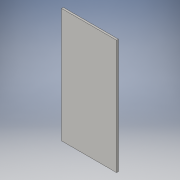
# Autodesk Inventor part: RaspberryBox_Backplate
Saved by Autodesk Inventor 2016 (Build 200138000, 138)
## iProperties
Created: 2016-12-27
Part Number: RaspberryBox_Backplate
Material: Generisch
Document SubType Name: Modeling
Designer: Moritz
Density: 1 g/cm^3
Appearance: Vorgabe
Author: Moritz
Autodesk Inventor part; units mm, degrees
ref_plane "YZ Plane" through (0, 0, 0) normal (1, 0, 0) x (0, 1, 0)
ref_plane "XZ Plane" through (0, 0, 0) normal (0, 1, 0) x (-1, 0, 0)
ref_plane "XY Plane" through (0, 0, 0) normal (0, 0, 1) x (1, 0, 0)
sketch "Skizze1" plane through (0, 0, 0) normal (0, 1, 0) x (-1, 0, 0)
  line L0 (-44, 91.5) -> (44, 91.5)
  line L1 (44, 91.5) -> (44, -91.5)
  line L2 (44, -91.5) -> (-44, -91.5)
  line L3 (-44, -91.5) -> (-44, 91.5)
  line L4 (-44, 91.5) -> (44, -91.5) construction
  line L5 (44, 91.5) -> (-44, -91.5) construction
  point P0 (0, 0)
  dimension "d0" = 88
  dimension "d1" = 183
  constraints: 12 end point, 2 midpoint, 2 parallel, 1 horizontal, 1 perpendicular
  measures "d0" distance of L1.end L2.end
  measures "d1" distance of L0.end L1.end
extrude "Extrusion1" add sketch "Skizze1" along normal blind 3
